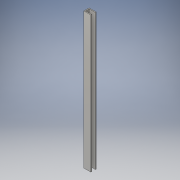
# Autodesk Inventor part: Small C Channel
Saved by Autodesk Inventor 2016 (Build 200138000, 138)
## iProperties
Created: 2016-11-17
Part Number: Small C Channel
Material: Aluminum 6061
Document SubType Name: Modeling
Designer: 17kressc
Density: 2.7 g/cm^3
Appearance: Aluminum - Polished
Mass: 32.8381 g
Surface Area: 161.895 cm^2
Volume: 12.1623 cm^3
Author: 17kressc
Autodesk Inventor part; units mm, degrees
ref_plane "YZ Plane" through (0, 0, 0) normal (1, 0, 0) x (0, 1, 0)
ref_plane "XZ Plane" through (0, 0, 0) normal (0, 1, 0) x (-1, 0, 0)
ref_plane "XY Plane" through (0, 0, 0) normal (0, 0, 1) x (1, 0, 0)
sketch "Sketch1" plane through (0, 0, 0) normal (0, 1, 0) x (-1, 0, 0)
  line L0 (0, 0) -> (12.7, 0)
  line L1 (12.7, 0) -> (12.7, -9.525)
  line L2 (12.7, -9.525) -> (0, -9.525)
  line L3 (0, -1.5875) -> (11.1125, -1.5875)
  line L4 (11.1125, -1.5875) -> (11.1125, -7.9375)
  line L5 (11.1125, -7.9375) -> (0, -7.9375)
  line L6 (0, -9.525) -> (0, -7.9375)
  line L7 (0, -1.5875) -> (0, 0)
  dimension "d0" = 12.7
  dimension "d1" = 9.525
  dimension "d2" = 6.35
  dimension "d3" = 1.5875
  dimension "d4" = 1.5875
  dimension "d5" = 1.5875
  constraints: 16 end point, 4 perpendicular, 3 parallel, 2 horizontal
  measures "d0" distance of L1.end L2.end
  measures "d1" distance of L0.end L1.end
  measures "d2" distance between parallel lines of L5 L3
  measures "d3" distance between parallel lines of L2 L5
  measures "d4" distance between parallel lines of L3 L0
  measures "d5" distance between parallel lines of L1 L4
extrude "Extrusion1" add sketch "Sketch1" along normal blind 241.3
body "Solid1"
